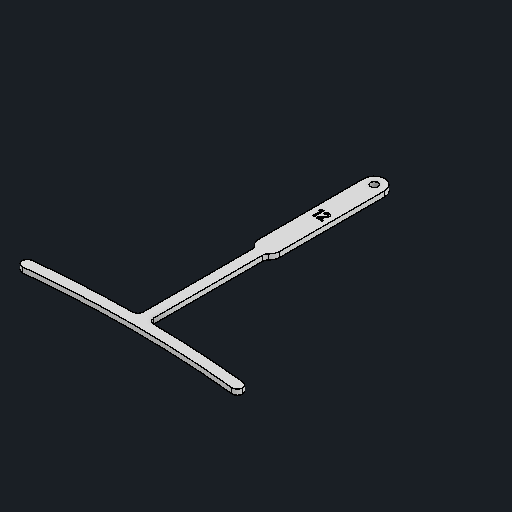
# Autodesk Inventor part: Understring Radius Gauge
Saved by Autodesk Inventor 2026.2 (Build 302298000, 298)
## iProperties
Created: 2026-03-05
Part Number: Understring Radius Gauge
Material: Generic
Document SubType Name: Modeling
Designer: JoshuaEah
Density: 1 g/cm^3
Appearance: Default
Author: JoshuaEah
Autodesk Inventor part; units mm, degrees
ref_plane "YZ Plane" through (0, 0, 0) normal (1, 0, 0) x (0, 1, 0)
ref_plane "XZ Plane" through (0, 0, 0) normal (0, 1, 0) x (-1, 0, 0)
ref_plane "XY Plane" through (0, 0, 0) normal (0, 0, 1) x (1, 0, 0)
sketch "Sketch1" plane through (0, 0, 0) normal (0, 1, 0) x (-1, 0, 0)
  arc A0 (-304.8, 0) -> (304.8, 0) centre (0, 0) ccw
  line L0 (0, 0) -> (304.8, 0) construction
  line L1 (0, 0) -> (304.8, 0) construction
  line L2 (0, 0) -> (-304.8, 0) construction
  arc A1 (-304.8, -3.175) -> (304.8, -3.175) centre (0, -3.175) ccw
  line L3 (0, -3.175) -> (304.8, -3.175) construction
  line L4 (0, -3.175) -> (304.8, -3.175) construction
  line L5 (0, -3.175) -> (-304.8, -3.175) construction
  line L6 (0, -304.8) -> (0, -381)
  line L7 (0, -381) -> (0, -342.9) construction
  line L8 (3.175, -377.825) -> (3.175, -346.075)
  line L9 (-3.175, -346.075) -> (-3.175, -377.825)
  arc A2 (-3.175, -377.825) -> (3.175, -377.825) centre (0, -377.825) ccw
  arc A3 (3.175, -346.075) -> (-3.175, -346.075) centre (0, -346.075) ccw
  line L10 (1.5875, -343.3254) -> (1.5875, -307.9709)
  line L11 (-1.5875, -343.3254) -> (-1.5875, -307.9709)
  line L12 (33.3375, -306.1464) -> (33.3375, -302.9714)
  line L13 (-33.3375, -306.1464) -> (-33.3375, -302.9714)
  line L14 (2.4621, -359.5082) -> (-2.4621, -359.5082) construction
  line L15 (-2.4621, -359.5082) -> (-2.4621, -364.3918) construction
  line L16 (-2.4621, -364.3918) -> (2.4621, -364.3918) construction
  line L17 (2.4621, -364.3918) -> (2.4621, -359.5082) construction
  line L18 (0.774, -363.4564) -> (0.774, -360.4084)
  line L19 (0.774, -360.4084) -> (1.2018, -360.4084)
  line L20 (1.2018, -360.4084) -> (1.2018, -362.9907)
  line L21 (1.2018, -362.9907) -> (1.6347, -362.724)
  line L22 (1.6347, -362.724) -> (1.6347, -363.1669)
  line L23 (1.6347, -363.1669) -> (1.2018, -363.4564)
  line L24 (1.2018, -363.4564) -> (0.774, -363.4564)
  line L25 (0.1271, -360.4084) -> (0.1271, -360.7809)
  line L26 (0.1271, -360.7809) -> (-0.935, -362.1979)
  spline S0 degree 2 poles (-0.935, -362.1979) (-1.0282, -362.3212) (-1.1288, -362.5805) (-1.1288, -362.6963) knots 0 0 0 1 2 2 2
  line L27 (-1.1288, -362.6963) -> (-1.1288, -362.6988)
  spline S1 degree 2 poles (-1.1288, -362.6988) (-1.1288, -362.8825) (-0.9149, -363.0839) (-0.7186, -363.0839) knots 0 0 0 1 2 2 2
  spline S2 degree 2 poles (-0.7186, -363.0839) (-0.5348, -363.0839) (-0.3008, -362.8649) (-0.2756, -362.6635) knots 0 0 0 1 2 2 2
  line L28 (-0.2756, -362.6635) -> (-0.2756, -362.661)
  line L29 (-0.2756, -362.661) -> (0.1649, -362.661)
  line L30 (0.1649, -362.661) -> (0.1649, -362.6635)
  spline S3 degree 2 poles (0.1649, -362.6635) (0.1095, -363.0562) (-0.3511, -363.4916) (-0.7161, -363.4916) knots 0 0 0 1 2 2 2
  spline S4 degree 2 poles (-0.7161, -363.4916) (-1.1263, -363.4916) (-1.5743, -363.0763) (-1.5743, -362.6963) knots 0 0 0 1 2 2 2
  line L31 (-1.5743, -362.6963) -> (-1.5743, -362.6938)
  spline S5 degree 2 poles (-1.5743, -362.6938) (-1.5743, -362.5327) (-1.4409, -362.1778) (-1.3201, -362.0167) knots 0 0 0 1 2 2 2
  line L32 (-1.3201, -362.0167) -> (-0.4392, -360.8161)
  line L33 (-0.4392, -360.8161) -> (-1.592, -360.8161)
  line L34 (-1.592, -360.8161) -> (-1.592, -360.4084)
  line L35 (-1.592, -360.4084) -> (0.1271, -360.4084)
  point P0 (0, -361.95)
  point P1 (0, -342.9)
  point P2 (0, -381)
  dimension "gaugeRadius" = 304.8
  dimension "d2" = 304.8
  dimension "d3" = 0
  dimension "d4" = 180
  dimension "d5" = 304.8
  dimension "d6" = 0
  dimension "d7" = 180
  dimension "d8" = 3.175
  dimension "d9" = 76.2
  dimension "d10" = 6.35
  dimension "d11" = 38.1
  dimension "d12" = 3.175
  dimension "d13" = 66.675
  dimension "d25" = 0.7129
  dimension "d26" = 0.7129
  dimension "d27" = 18.3167
  dimension "d28" = 18.3167
  constraints: 30 end point, 17 point on circle, 4 centre point, 4 symmetric about line, 4 tangent, 3 vertical, 2 collinear, 2 horizontal, 2 midpoint, 2 point on line, 1 coincident, 1 parallel, 1 vertical alignment, 3 other
  measures "d2" radius of A0
  measures "d3" distance between parallel lines of L0 L1
  measures "d4" angle of L2 L0
  measures "d5" radius of A1
  measures "d6" distance between parallel lines of L3 L4
  measures "d7" angle of L5 L3
  measures "d8" distance of L0.start L3.start
  measures "d9" distance of L6.start L6.end
  measures "d10" diameter of A3
  measures "d11" distance of point (0, -342.9) point (0, -381)
  measures "d12" diameter of L10 L6
  measures "d13" diameter of L12 L6
  measures "d25" distance between parallel lines of L8 L17
  measures "d26" distance between parallel lines of L9 L15
  measures "d27" distance from line of A3.centre L16
  measures "d28" distance from line of L14 A2.centre
extrude "Extrusion1" add sketch "Sketch1" against normal blind 1.5875 contours A0 L6 A1 L13 | A0 L12 A1 L6 | L6 A3 L11 A1 | A1 L10 A3 L6 | A3 L8 A2 L6 S3 L30 L29 L26 L25 L35 | L6 L35 L34 L33 L32 S5 L31 S4 S3 A2 L9 A3 | L35 L25 L26 L6 | L6 L26 S0 L27 S1 S2 L28 L29 S3 S4 L31 S5 L32 L33 L34 L35 | L6 L29 L28 S2 S1 L27 S0 L26 | L29 L30 S3 L6 | L18 L19 L20 L21 L22 L23 L24
fillet "Fillet1" radius 1.5875 4 edges at (-33.3375, -0.7937, -302.9714) (-33.3375, -0.7937, -306.1464) (33.3375, -0.7937, -302.9714) (33.3375, -0.7937, -306.1464)
fillet "Fillet2" radius 1.5875 4 edges at (1.5875, -0.7937, -307.9709) (-1.5875, -0.7937, -307.9709) (1.5875, -0.7937, -343.3254) (-1.5875, -0.7937, -343.3254)
hole "Hole1" at (0, 0, -377.825) direction (0, 1, 0) diameter 2.2606 end through all start extended yes clearance for "Flat Head Machine Screw (82)" size "#2" standard "Ansi Unified Screw Threads"
emboss "Emboss1" sketch "Sketch1" operation cut depth 0.0762 direction (0, -1, 0) contours L35 L25 L26 L6 | L6 L26 S0 L27 S1 S2 L28 L29 S3 S4 L31 S5 L32 L33 L34 L35 | L29 L30 S3 L6 | L18 L19 L20 L21 L22 L23 L24
sketch "LASERCUT" plane through (0, 0, 0) normal (0, 1, 0) x (1, 0, 0)
  line L0 (-0.1649, 362.661) -> (-0.1649, 362.6635) projected
  line L1 (1.5743, 362.6963) -> (1.5743, 362.6938) projected
  line L2 (1.3201, 362.0167) -> (0.4392, 360.8161) projected
  line L3 (0.4392, 360.8161) -> (1.592, 360.8161) projected
  line L4 (1.592, 360.8161) -> (1.592, 360.4084) projected
  line L5 (1.592, 360.4084) -> (-0.1271, 360.4084) projected
  line L6 (-0.1271, 360.4084) -> (-0.1271, 360.7809) projected
  line L7 (-0.1271, 360.7809) -> (0.935, 362.1979) projected
  line L8 (1.1288, 362.6963) -> (1.1288, 362.6988) projected
  line L9 (0.2756, 362.6635) -> (0.2756, 362.661) projected
  line L10 (0.2756, 362.661) -> (-0.1649, 362.661) projected
  line L11 (-0.774, 363.4564) -> (-0.774, 360.4084) projected
  line L12 (-0.774, 360.4084) -> (-1.2018, 360.4084) projected
  line L13 (-1.2018, 360.4084) -> (-1.2018, 362.9907) projected
  line L14 (-1.2018, 362.9907) -> (-1.6347, 362.724) projected
  line L15 (-1.6347, 362.724) -> (-1.6347, 363.1669) projected
  line L16 (-1.6347, 363.1669) -> (-1.2018, 363.4564) projected
  line L17 (-1.2018, 363.4564) -> (-0.774, 363.4564) projected
  circle A0 centre (0, 377.825) radius 1.1303 projected
  arc A1 (33.3375, 304.738) -> (31.9163, 306.2994) centre (31.7501, 304.7206) ccw projected
  arc A2 (31.9163, 306.2994) -> (3.1585, 307.9586) centre (0, 3.175) ccw projected
  arc A3 (1.5875, 309.546) -> (3.1585, 307.9586) centre (3.175, 309.546) ccw projected
  line L18 (1.5875, 309.546) -> (1.5875, 342.5252) projected
  arc A4 (2.1167, 343.7085) -> (1.5875, 342.5252) centre (3.175, 342.5252) ccw projected
  arc A5 (2.1167, 343.7085) -> (3.175, 346.075) centre (0, 346.075) ccw projected
  line L19 (3.175, 346.075) -> (3.175, 377.825) projected
  arc A6 (3.175, 377.825) -> (-3.175, 377.825) centre (0, 377.825) ccw projected
  line L20 (-3.175, 377.825) -> (-3.175, 346.075) projected
  arc A7 (-3.175, 346.075) -> (-2.1167, 343.7085) centre (0, 346.075) ccw projected
  arc A8 (-1.5875, 342.5252) -> (-2.1167, 343.7085) centre (-3.175, 342.5252) ccw projected
  line L21 (-1.5875, 342.5252) -> (-1.5875, 309.546) projected
  arc A9 (-3.1585, 307.9586) -> (-1.5875, 309.546) centre (-3.175, 309.546) ccw projected
  arc A10 (-3.1585, 307.9586) -> (-31.9163, 306.2994) centre (0, 3.175) ccw projected
  arc A11 (-31.9163, 306.2994) -> (-33.3375, 304.738) centre (-31.7501, 304.7206) ccw projected
  arc A12 (-33.3375, 304.738) -> (-31.5855, 303.159) centre (-31.75, 304.738) ccw projected
  arc A13 (31.5855, 303.159) -> (-31.5855, 303.159) centre (0, 0) ccw projected
  arc A14 (31.5855, 303.159) -> (33.3375, 304.738) centre (31.75, 304.738) ccw projected
  constraints: 6 other
equation "\"gaugeRadius\" = 304.8"
equation "\"d2\" = gaugeRadius"
equation "\"d5\" = gaugeRadius"
equation "\"d8\" = gaugeHeight"
equation "\"d9\" = handleLength"
equation "\"d10\" = gripWidth"
equation "\"d11\" = gripLength"
equation "\"d12\" = 0.5 * gripWidth"
equation "\"d13\" = gaugeWidth"
equation "\"d26\" = d25"
equation "\"d28\" = d27"
equation "\"d16\" = 0.5 * gaugeHeight"
equation "\"d17\" = 0.25 * gripWidth"
equation "\"gaugeHeight\" = 3.175"
equation "\"gaugeWidth\" = 66.675"
equation "\"handleLength\" = 76.2"
equation "\"gripWidth\" = 6.35"
equation "\"gripLength\" = 38.1"
body "Solid1"
